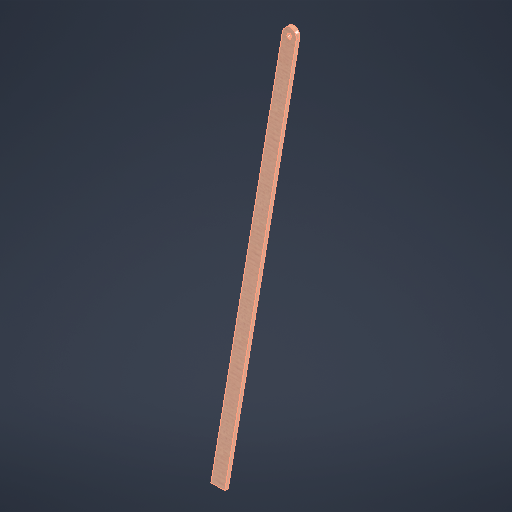
# Autodesk Inventor part: UPRIGHTS_TREBUCHET
Saved by Autodesk Inventor 2026.2 (Build 302298010, 298A)
## iProperties
Created: 2026-02-18
Part Number: UPRIGHTS_TREBUCHET
Material: Wood (Oak)
Document SubType Name: Modeling
Designer: 4aida
Density: 0.76 g/cm^3
Appearance: White Oak - Natural Medium Gloss
Author: 4aida
Autodesk Inventor part; units mm, degrees
ref_plane "YZ Plane" through (0, 0, 0) normal (1, 0, 0) x (0, 1, 0)
ref_plane "XZ Plane" through (0, 0, 0) normal (0, 1, 0) x (-1, 0, 0)
ref_plane "XY Plane" through (0, 0, 0) normal (0, 0, 1) x (1, 0, 0)
sketch "Sketch1" plane through (0, 0, 0) normal (1, 0, 0) x (0, 1, 0)
  line L0 (0, 4.8581) -> (0, -4.8581)
  line L1 (0, 4.8581) -> (1000, -196.5631)
  line L2 (1000, -196.5631) -> (1000, -206.2794)
  line L3 (1000, -206.2794) -> (0, -4.8581)
  point P0 (0, 0)
  point P1 (0, 0)
  dimension "d0" = 9.525
  dimension "d1" = 1000
  dimension "d9" = 211.1375
  dimension "d10" = 78.612
  constraints: 8 end point, 2 parallel, 1 coincident, 1 midpoint, 1 vertical
  measures "d0" distance between parallel lines of L3 L1
  measures "d1" distance between parallel lines of L0 L2
  measures "d9" vertical distance of L2.end L0.start
  measures "d10" angle of L3 L0
extrude "Extrusion1" add sketch "Sketch1" along normal mid plane 38.1
sketch "Sketch2" plane through (0, 0, 0) normal (0, 0, 1) x (1, 0, 0)
  circle A0 centre (0, 980.95) radius 6.35
  circle A1 centre (0, 980.95) radius 19.05
  line L0 (19.05, 1000) -> (19.05, 0) projected
  line L1 (-19.05, 1000) -> (19.05, 1000) projected
  line L2 (-19.05, 1000) -> (-19.05, 980.95)
  point P0 (0, 0)
  point P1 (0, 1000)
  point P2 (19.05, 980.95)
  dimension "d5" = 38.1
  dimension "d6" = 12.7
  constraints: 2 end point, 2 vertical, 1 centre point, 1 coincident, 1 horizontal, 3 other
  measures "d6" diameter of A0
extrude "Extrusion2" cut sketch "Sketch2" along normal through all both and the other way through all contours A0 | L2 L1 A1 | A1 L1 L0
body "Solid1"
